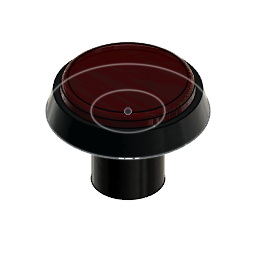
button_v1 (Autodesk Fusion 360 design; units mm, degrees)
Autodesk Fusion 360 part; units mm, degrees
sketch "Sketch1" plane through (0, 0, 0) normal (0, 0, 1) x (1, 0, 0)
  circle A0 centre (0, 0) radius 13.5
  circle A1 centre (0, 0) radius 30
  dimension "d1" = 27
  dimension "d2" = 60
  constraint coincident A0.centre A1.centre
  measures "d1" diameter of A0
  measures "d2" diameter of A1
extrude "Extrude1" add sketch "Sketch1" against normal blind 30 contours A0 makes body 1
extrude "Extrude2" add sketch "Sketch1" along normal blind 10 draft -15 contours A0 | A1 bodies 1
sketch "Sketch2" plane through (0, 0, 10) normal (0, 0, 1) x (-1, 0, 0)
  circle A0 centre (0, 0) radius 27.3205
  circle A1 centre (0, 0) radius 25
  constraint concentric A0 A1
extrude "Extrude3" add sketch "Sketch2" along normal blind 5 draft -10 separate body contours A1 makes body 2
fillet "Fillet1" radius 2.5 1 edges at (22.4862, -8.7216, 15) on bodies 2
